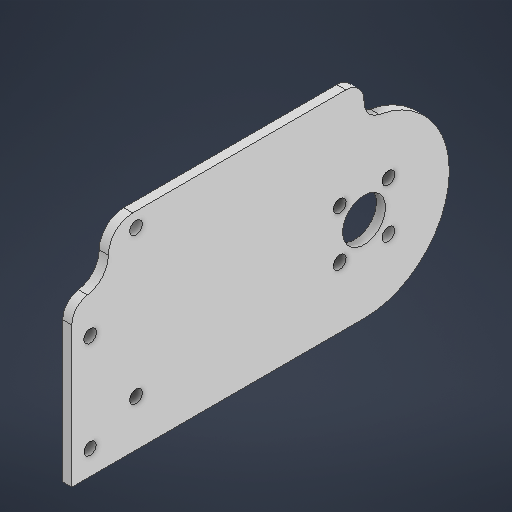
# Autodesk Inventor part: EndEffectorStage1Plate
Saved by Autodesk Inventor 2025 (Build 290162000, 162)
## iProperties
Created: 2024-04-08
Part Number: EndEffectorStage1Plate
Material: Generic
Document SubType Name: Modeling
Designer: avsar
Density: 1 g/cm^3
Appearance: Default
Author: avsar
Autodesk Inventor part; units mm, degrees
ref_plane "YZ Plane" through (0, 0, 0) normal (1, 0, 0) x (0, 1, 0)
ref_plane "XZ Plane" through (0, 0, 0) normal (0, 1, 0) x (-1, 0, 0)
ref_plane "XY Plane" through (0, 0, 0) normal (0, 0, 1) x (1, 0, 0)
sketch "Sketch1" plane through (0, 0, 0) normal (1, 0, 0) x (0, 1, 0)
  arc A0 (-28, 0) -> (28, 0) centre (0, 0) ccw
  line L0 (-28, 0) -> (28, 0) construction
  line L1 (28, 0) -> (28, 96)
  line L2 (28, 96) -> (-28, 96)
  line L3 (-28, 96) -> (-28, 0)
  circle A1 centre (0, 0) radius 7.05
  circle A2 centre (8, 8) radius 2.1
  circle A3 centre (-8, 8) radius 2.1
  circle A4 centre (-8, -8) radius 2.1
  circle A5 centre (8, -8) radius 2.1
  circle A6 centre (12, 90) radius 2.1
  line L4 (0, 96) -> (0, 0) construction
  circle A7 centre (-20, 90) radius 2
  dimension "d0" = 28
  dimension "d1" = 96
  dimension "d2" = 14.1
  dimension "d3" = 4.2
  dimension "d4" = 8
  dimension "d5" = 8
  dimension "d8" = 360
  dimension "d10" = 4.2
  dimension "d11" = 12
  dimension "d12" = 6
  dimension "d43" = 4
  dimension "d44" = 32
  constraints: 10 end point, 8 centre point, 2 coincident, 2 horizontal alignment, 2 midpoint, 2 parallel, 2 point on circle, 1 horizontal, 1 perpendicular, 1 vertical, 9 other
  measures "d0" radius of A0
  measures "d1" distance of L0.end L1.end
  measures "d2" diameter of A1
  measures "d3" diameter of A2
  measures "d4" horizontal distance of L4.end A2.centre
  measures "d5" horizontal distance of point (0, 0) A2.centre
  measures "d10" diameter of A6
  measures "d11" horizontal distance of A6.centre point (0, 0)
  measures "d12" distance from line of L2 A6.centre
  measures "d43" diameter of A7
  measures "d44" distance of A6.centre A7.centre
extrude "Extrusion1" add sketch "Sketch1" along normal blind 3
sketch "Sketch2" plane through (3, 0, 0) normal (1, 0, 0) x (0, 0, -1)
  line L0 (-74.9, 35.5) -> (-74.9, -13) construction
  line L1 (-74.9, -13) -> (-74.9, 0) construction
  line L2 (-77.4, 35.25) -> (-72.4, 35.25) construction
  line L3 (-72.4, 35.25) -> (-72.4, -12.75) construction
  line L4 (-72.4, -12.75) -> (-77.4, -12.75) construction
  line L5 (-77.4, -12.75) -> (-77.4, 35.25) construction
  line L6 (-77.4, 35.25) -> (-72.4, -12.75) construction
  line L7 (-72.4, 35.25) -> (-77.4, -12.75) construction
  line L8 (0, 28) -> (-96, 28) projected
  line L9 (-96, 28) -> (-96, 40)
  line L10 (-96, 40) -> (0, 40)
  line L11 (0, 40) -> (0, 28)
  circle A0 centre (-74.9, 35.25) radius 2.1
  circle A1 centre (-74.9, -12.75) radius 2.1
  circle A2 centre (-90, 12) radius 2.1 projected
  point P0 (0, 0)
  point P1 (-74.9, 11.25)
  dimension "d17" = 48.5
  dimension "d18" = 13
  dimension "d19" = 5
  dimension "d20" = 48
  dimension "d22" = 12
  dimension "d24" = 4.2
  dimension "d31" = 4.2
  dimension "d34" = 15.1
  constraints: 22 end point, 5 midpoint, 3 perpendicular, 2 centre point, 2 parallel, 2 vertical, 1 horizontal, 1 horizontal alignment, 1 point on line
  measures "d17" distance of L0.start L0.end
  measures "d18" distance of L0.end L1.end
  measures "d19" distance of L3.end L4.end
  measures "d20" distance of L2.end L3.end
  measures "d22" distance of L8.end L9.end
  measures "d24" diameter of A0
  measures "d31" diameter of A1
  measures "d34" horizontal distance of A2.centre L0.start
extrude "Extrusion2" add sketch "Sketch2" against normal up to surface (3 mm away) contours L8 L9 L10 L11
fillet "Fillet1" radius 6 1 edges at (1.5, 28, 0)
fillet "Fillet2" radius 6 1 edges at (1.5, 40, 0)
extrude "Extrusion4" cut sketch "Sketch2" against normal through all contours A1
sketch "Sketch3" plane through (3, 0, 0) normal (1, 0, 0) x (0, 0, -1)
  line L0 (-96, -28) -> (-96, 40) projected
  line L1 (-6, 40) -> (-96, 40) projected
  line L2 (-96, 24) -> (-84, 24)
  line L3 (-84, 24) -> (-84, 40)
  point P0 (0, 0)
  dimension "d37" = 12
  dimension "d38" = 16
  constraints: 4 end point, 2 point on line, 1 horizontal, 1 perpendicular
  measures "d37" distance of L2.start L2.end
  measures "d38" distance of L2.end L3.end
extrude "Extrusion5" cut sketch "Sketch3" against normal through all
fillet "Fillet3" radius 8 2 edges at (1.5, 24, 84) (1.5, 40, 84)
fillet "Fillet4" radius 6 1 edges at (1.5, 24, 96)
body "Solid1"
